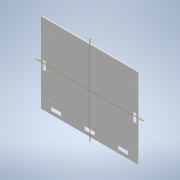
# Autodesk Inventor part: electronic_plate_long_side
Saved by Autodesk Inventor 2021.1 (Build 251245010, 245A)
## iProperties
Created: 2023-01-21
Part Number: electronic_plate_long_side
Material: Типовые
Document SubType Name: Modeling
Designer: zmoze
Density: 1 g/cm^3
Appearance: По умолчанию
Author: zmoze
Autodesk Inventor part; units mm, degrees
ref_plane "YZ Plane" through (0, 0, 0) normal (1, 0, 0) x (0, 1, 0)
ref_plane "XZ Plane" through (0, 0, 0) normal (0, 1, 0) x (-1, 0, 0)
ref_plane "XY Plane" through (0, 0, 0) normal (0, 0, 1) x (1, 0, 0)
sketch "Эскиз1" plane through (0, 0, 0) normal (0, 0, 1) x (1, 0, 0)
  line L0 (-145, 120) -> (145, 120)
  line L1 (145, 120) -> (145, -120)
  line L2 (145, -120) -> (-145, -120)
  line L3 (-145, -120) -> (-145, 120)
  line L4 (-145, 120) -> (145, -120) construction
  line L5 (145, 120) -> (-145, -120) construction
  point P0 (0, 0)
  dimension "d0" = 290
  dimension "d1" = 240
  constraints: 12 end point, 2 midpoint, 2 parallel, 1 horizontal, 1 perpendicular
  measures "d0" distance of L0.start L0.end
  measures "d1" distance of L0.end L1.end
extrude "Выдавливание1" add sketch "Эскиз1" along normal blind 3
sketch "Эскиз2" plane through (0, 0, 3) normal (0, 0, 1) x (1, 0, 0)
  line L0 (-5, 95) -> (5, 95)
  line L1 (145, 120) -> (-145, 120) projected
  line L2 (0, 168) -> (0, -168) projected
  line L3 (-101.423, -89.3301) -> (-106.423, -80.6699)
  line L4 (106.423, -80.6699) -> (101.423, -89.3301)
  point P0 (0, 0)
  point P1 (0, 95)
  point P2 (0, -25)
  point P3 (-103.923, -85)
  point P4 (103.923, -85)
  dimension "d4" = 25
  dimension "d5" = 10
  dimension "d8" = 360
  dimension "d10" = 120
  constraints: 6 end point, 2 point on line, 1 horizontal, 1 midpoint, 13 other
  measures "d4" distance between parallel lines of L0 L1
  measures "d5" distance of L0.start L0.end
  measures "d10" distance from line of point (0, -25) L0
sketch "Эскиз4" plane through (0, 0, 0) normal (0, 0, -1) x (-1, 0, 0)
  line L0 (130, -15.5) -> (130, 9.5) projected
  line L1 (130, 9.5) -> (140, 9.5) projected
  line L2 (140, 9.5) -> (140, -15.5) projected
  line L3 (140, -15.5) -> (130, -15.5) projected
  line L4 (-15, -100) -> (15, -100) projected
  line L5 (15, -100) -> (15, -110) projected
  line L6 (15, -110) -> (-15, -110) projected
  line L7 (-15, -110) -> (-15, -100) projected
  line L8 (115, -100) -> (115, -110) projected
  line L9 (115, -110) -> (85, -110) projected
  line L10 (85, -110) -> (85, -100) projected
  line L11 (85, -100) -> (115, -100) projected
  line L12 (-130, -15.5) -> (-140, -15.5) projected
  line L13 (-140, -15.5) -> (-140, 9.5) projected
  line L14 (-140, 9.5) -> (-130, 9.5) projected
  line L15 (-130, 9.5) -> (-130, -15.5) projected
  circle A0 centre (120, 79) radius 1.5 projected
  circle A1 centre (-120, -85) radius 1.5 projected
  circle A2 centre (120, -85) radius 1.5 projected
  line L16 (-85, -100) -> (-85, -110) projected
  line L17 (-85, -110) -> (-115, -110) projected
  line L18 (-115, -110) -> (-115, -100) projected
  line L19 (-115, -100) -> (-85, -100) projected
  circle A3 centre (-120, 79) radius 1.5 projected
  line L20 (150, 119) -> (-150, 119) projected
  line L21 (-150, 119) -> (-150, -125) projected
  line L22 (-150, -125) -> (150, -125) projected
  line L23 (150, -125) -> (150, 119) projected
  point P0 (0, 0)
extrude "Выдавливание3" cut sketch "Эскиз4" against normal blind 10 contours L0 L1 L2 L3 | L4 L5 L6 L7 | L8 L9 L10 L11 | L12 L13 L14 L15 | A0 | A1 | A2 | L16 L17 L18 L19 | A3
